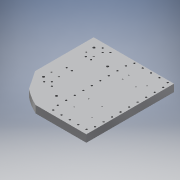
# Autodesk Inventor part: Base Plate Mk 2
Saved by Autodesk Inventor 2017 (Build 210142000, 142)
## iProperties
Created: 2016-12-06
Part Number: Base Plate Mk 2
Material: Aluminum 6061
Document SubType Name: Modeling
Designer: qupec
Density: 2.7 g/cm^3
Appearance: Aluminum - Flat
Mass: 681.535 g
Surface Area: 529.714 cm^2
Volume: 252.42 cm^3
Author: qupec
Autodesk Inventor part; units mm, degrees
ref_plane "YZ Plane" through (0, 0, 0) normal (1, 0, 0) x (0, 1, 0)
ref_plane "XZ Plane" through (0, 0, 0) normal (0, 1, 0) x (-1, 0, 0)
ref_plane "XY Plane" through (0, 0, 0) normal (0, 0, 1) x (1, 0, 0)
sketch "Sketch1" plane through (0, 0, 0) normal (0, 1, 0) x (-1, 0, 0)
  line L0 (69.85, 76.2) -> (-69.85, 76.2)
  line L1 (-69.85, 76.2) -> (-69.85, -76.2)
  line L2 (-69.85, -76.2) -> (69.85, -76.2)
  line L3 (69.85, -76.2) -> (69.85, 76.2)
  point P0 (0, 0)
  dimension "d0" = 152.4
  dimension "d1" = 139.7
  dimension "d2" = 69.85
  dimension "d3" = 76.2
  constraints: 8 end point, 2 parallel, 1 horizontal, 1 perpendicular
  measures "d0" distance of L2.end L0.start
  measures "d1" distance of L0.start L0.end
  measures "d2" distance from line of point (0, 0) L1
  measures "d3" distance from line of point (0, 0) L0
extrude "Extrusion1" add sketch "Sketch1" along normal blind 12.7
fillet "Fillet1" [suppressed]
sketch "Sketch7" plane through (0, 12.7, 0) normal (0, 1, 0) x (1, 0, 0)
  arc A0 (-69.85, -37.0366) -> (-18.2851, -76.2) centre (46.0045, 61.976) ccw
  line L0 (69.85, 76.2) -> (-69.85, 76.2) projected
  line L1 (69.85, -76.2) -> (69.85, 76.2) projected
  line L2 (-69.85, 76.2) -> (-69.85, -76.2) projected
  line L3 (-69.85, -76.2) -> (69.85, -76.2) projected
  line L4 (-69.85, 76.2) -> (-69.85, -76.2) projected
  arc A1 (-18.2851, -76.2) -> (-69.85, -37.0366) centre (46.0045, 61.976) ccw
  point P0 (0, 0)
  point P1 (76.2, -60.325)
  point P2 (73.025, -60.325)
  point P3 (73.025, 63.5)
  point P4 (73.025, 60.325)
  point P5 (-73.025, 63.5)
  point P6 (76.2, 60.325)
  point P7 (73.025, -63.5)
  point P8 (-76.2, 60.325)
  point P9 (-80.9955, -22.2663)
  dimension "d46" = 304.8
  dimension "d47" = 14.224
  dimension "d48" = 23.8455
  constraints: 5 point on circle, 2 centre point, 7 other
  measures "d46" diameter of A0
sketch "Sketch8" plane through (0, 12.7, 0) normal (0, 1, 0) x (1, 0, 0)
  circle A0 centre (-47.526, 7.0319) radius 1.4224 projected
  circle A1 centre (-47.526, 7.0319) radius 1.4224 projected
  circle A2 centre (-38.506, 7.0319) radius 1.4224 projected
  line L0 (-33.996, 3.9778) -> (-52.036, 3.9778) projected
  line L1 (-33.996, 10.086) -> (-33.996, 3.9778) projected
  line L2 (-33.996, 10.086) -> (-52.036, 10.086) projected
  line L3 (-52.036, 3.9778) -> (-52.036, 10.086) projected
  circle A3 centre (-47.526, 40.2937) radius 1.4224 projected
  circle A4 centre (-38.506, 40.2937) radius 1.4224 projected
  line L4 (-33.996, 37.2396) -> (-52.036, 37.2396) projected
  line L5 (-33.996, 43.3478) -> (-33.996, 37.2396) projected
  line L6 (-33.996, 43.3478) -> (-52.036, 43.3478) projected
  line L7 (-52.036, 37.2396) -> (-52.036, 43.3478) projected
  circle A5 centre (2.54, -39.6875) radius 3.175 construction
  circle A6 centre (2.54, 12.7127) radius 3.175 construction
  circle A7 centre (2.54, 65.1129) radius 3.175 construction
  circle A8 centre (68.58, 65.1129) radius 3.175 construction
  circle A9 centre (68.58, 12.7127) radius 3.175 construction
  circle A10 centre (68.58, -39.6875) radius 3.175 construction
  circle A11 centre (-32.4275, -33.782) radius 1.4224 projected
  circle A12 centre (-39.1585, -27.051) radius 1.4224 projected
  circle A13 centre (-45.8895, -33.782) radius 1.4224 projected
  circle A14 centre (-45.8895, 67.818) radius 1.4224 projected
  circle A15 centre (-39.1585, 61.087) radius 1.4224 projected
  circle A16 centre (-32.4275, 67.818) radius 1.4224 projected
extrude "Extrusion9" cut sketch "Sketch8" against normal through all contours A0 | A2 | A3 | A4 | A11 | A12 | A13 | A14 | A15 | A16
extrude "Extrusion11" cut sketch "Sketch7" against normal through all contours A0 L3 L2
sketch "Sketch10" plane through (0, 12.7, 0) normal (0, 1, 0) x (1, 0, 0)
  circle A0 centre (62.611, 72.39) radius 1.4732 projected
  arc A1 (-69.85, -37.0366) -> (-18.2851, -76.2) centre (46.0045, 61.976) ccw projected
  line L0 (-18.2851, -76.2) -> (69.85, -76.2) projected
  line L1 (69.85, -76.2) -> (69.85, 76.2) projected
  line L2 (69.85, 76.2) -> (-69.85, 76.2) projected
  line L3 (-69.85, 76.2) -> (-69.85, -37.0366) projected
  circle A2 centre (-47.526, 40.2937) radius 1.4224 projected
  circle A3 centre (-47.526, 7.0319) radius 1.4224 projected
  circle A4 centre (-38.506, 7.0319) radius 1.4224 projected
  circle A5 centre (-38.506, 40.2937) radius 1.4224 projected
  circle A6 centre (33.655, 72.39) radius 1.4732 projected
  circle A7 centre (48.133, 72.39) radius 1.4732 projected
  circle A8 centre (19.177, 72.39) radius 1.4732 projected
  circle A9 centre (4.699, 72.39) radius 1.4732 projected
  circle A10 centre (62.611, -68.58) radius 1.4732 projected
  circle A11 centre (48.133, -68.58) radius 1.4732 projected
  circle A12 centre (33.655, -68.58) radius 1.4732 projected
  circle A13 centre (19.177, -68.58) radius 1.4732 projected
  circle A14 centre (4.699, -68.58) radius 1.4732 projected
  point P0 (0, 0)
extrude "Extrusion13" cut sketch "Sketch10" against normal through all contours A0 | A6 | A7 | A8 | A9 | A10 | A11 | A12 | A13 | A14
sketch "Sketch11" plane through (0, 12.7, 0) normal (0, 1, 0) x (1, 0, 0)
  circle A0 centre (19.177, 72.39) radius 1.4732 projected
  circle A1 centre (48.133, 72.39) radius 1.4732 projected
  circle A2 centre (62.611, -68.58) radius 1.4732 projected
  circle A3 centre (33.655, -68.58) radius 1.4732 projected
  circle A4 centre (4.699, -68.58) radius 1.4732 projected
  circle A5 centre (1.27, -42.545) radius 1.4732 projected
  circle A6 centre (1.27, -12.9117) radius 1.4732 projected
  circle A7 centre (1.27, 16.7217) radius 1.4732 projected
  circle A8 centre (1.27, 46.355) radius 1.4732 projected
  circle A9 centre (66.04, 61.1717) radius 1.4732 projected
  circle A10 centre (66.04, 31.5383) radius 1.4732 projected
  circle A11 centre (66.04, 1.905) radius 1.4732 projected
  circle A12 centre (66.04, -27.7283) radius 1.4732 projected
  circle A13 centre (66.04, -57.3617) radius 1.4732 projected
  circle A14 centre (66.04, -42.545) radius 1.4732 projected
  circle A15 centre (66.04, -12.9117) radius 1.4732 projected
  circle A16 centre (66.04, 16.7217) radius 1.4732 projected
  circle A17 centre (66.04, 46.355) radius 1.4732 projected
  circle A18 centre (1.27, 61.1717) radius 1.4732 projected
  circle A19 centre (1.27, 31.5383) radius 1.4732 projected
  circle A20 centre (1.27, 1.905) radius 1.4732 projected
  circle A21 centre (1.27, -27.7283) radius 1.4732 projected
  circle A22 centre (1.27, -57.3617) radius 1.4732 projected
  circle A23 centre (19.177, -68.58) radius 1.4732 projected
  circle A24 centre (48.133, -68.58) radius 1.4732 projected
  circle A25 centre (62.611, 72.39) radius 1.4732 projected
  circle A26 centre (33.655, 72.39) radius 1.4732 projected
  circle A27 centre (4.699, 72.39) radius 1.4732 projected
  line L0 (0.635, -72.39) -> (66.675, -72.39) projected
  line L1 (69.85, -69.215) -> (69.85, 73.025) projected
  line L2 (66.675, 76.2) -> (0.635, 76.2) projected
  line L3 (-2.54, 73.025) -> (-2.54, -69.215) projected
  arc A28 (59.055, 62.23) -> (55.88, 65.405) centre (55.88, 62.23) ccw projected
  line L4 (59.055, -58.42) -> (59.055, 62.23) projected
  arc A29 (55.88, -61.595) -> (59.055, -58.42) centre (55.88, -58.42) ccw projected
  line L5 (11.43, -61.595) -> (55.88, -61.595) projected
  arc A30 (8.255, -58.42) -> (11.43, -61.595) centre (11.43, -58.42) ccw projected
  line L6 (8.255, 62.23) -> (8.255, -58.42) projected
  arc A31 (11.43, 65.405) -> (8.255, 62.23) centre (11.43, 62.23) ccw projected
  line L7 (55.88, 65.405) -> (11.43, 65.405) projected
  arc A32 (69.85, 73.025) -> (66.675, 76.2) centre (66.675, 73.025) ccw projected
  arc A33 (0.635, 76.2) -> (-2.54, 73.025) centre (0.635, 73.025) ccw projected
  arc A34 (-2.54, -69.215) -> (0.635, -72.39) centre (0.635, -69.215) ccw projected
  arc A35 (66.675, -72.39) -> (69.85, -69.215) centre (66.675, -69.215) ccw projected
  point P0 (0, 0)
  point P1 (52.705, -61.595)
extrude "Extrusion14" cut sketch "Sketch11" against normal through all contours A5 | A6 | A7 | A8 | A9 | A10 | A11 | A12 | A13 | A14 | A15 | A16 | A17 | A18 | A19 | A20 | A21 | A22 | A25
sketch "Sketch14" plane through (0, 0, 0) normal (0, -1, 0) x (1, 0, 0)
  line L0 (69.85, -76.2) -> (-69.85, -76.2) projected
  line L1 (-18.2851, 76.2) -> (69.85, 76.2) projected
  circle A0 centre (4.699, -72.39) radius 1.4732 projected
  circle A1 centre (-32.4275, -67.818) radius 1.4224 projected
  point P0 (0, 0)
  point P1 (-13.8643, 44.45)
  point P2 (-13.8643, -44.45)
  dimension "d79" = 44.45
  dimension "d80" = 152.4
  dimension "d81" = 44.45
  dimension "d82" = 37.1265
  dimension "d83" = 18.5633
  dimension "d84" = 18.5633
  measures "d79" vertical distance of point (0, 0) point (-13.864, 44.45)
  measures "d80" distance between parallel lines of L0 L1
  measures "d81" vertical distance of point (-13.864, -44.45) point (0, 0)
  measures "d82" horizontal distance of A0.centre A1.centre
  measures "d83" horizontal distance of A1.centre point (-13.864, -44.45)
  measures "d84" horizontal distance of A1.centre point (-13.864, 44.45)
hole "Hole2" at (-13.8643, 0, 44.45) at (-13.8643, 0, -44.45) direction (0, 1, 0) diameter 3.9624 end through all thread size "10-32 UNF" class "2B" standard "ANSI Unified Screw Threads"
sketch "Sketch15" plane through (0, 0, 0) normal (0, -1, 0) x (1, 0, 0)
  circle A0 centre (-13.8643, 44.45) radius 1.9812 projected
  circle A1 centre (-13.8643, -44.45) radius 1.9812 projected
  circle A2 centre (66.04, -31.5383) radius 1.4732 projected
  circle A3 centre (1.27, -31.5383) radius 1.4732 projected
  circle A4 centre (1.27, 42.545) radius 1.4732 projected
  point P0 (0, 0)
  point P1 (33.655, -44.45)
  point P2 (33.655, 44.45)
  point P3 (33.655, 0)
  dimension "d92" = 44.45
  dimension "d93" = 44.45
  dimension "d94" = 44.45
  dimension "d95" = 44.45
  dimension "d96" = 64.77
  dimension "d97" = 32.385
  dimension "d98" = 32.385
  dimension "d222" = 32.385
  dimension "d223" = 44.45
  measures "d92" vertical distance of point (0, 0) point (33.655, 44.45)
  measures "d93" vertical distance of point (0, 0) A0.centre
  measures "d94" vertical distance of point (0, 0) A1.centre
  measures "d95" vertical distance of point (33.655, -44.45) point (0, 0)
  measures "d96" distance between centres of A2 A3
  measures "d97" horizontal distance of A3.centre point (33.655, -44.45)
  measures "d98" horizontal distance of point (33.655, 44.45) A4.centre
  measures "d222" horizontal distance of A4.centre point (33.655, 0)
  measures "d223" distance of point (33.655, -44.45) point (33.655, 0)
hole "Hole3" at (33.655, 0, -44.45) at (33.655, 0, 44.45) at (33.655, 0, 0) direction (0, 1, 0) diameter 3.9624 depth 9.525 thread size "10-32 UNF" class "2B" standard "ANSI Unified Screw Threads"
thread "Thread3" size "5-40 UNC" class "2B" standard "ANSI Unified Screw Threads" full length
thread "Thread4" size "5-40 UNC" class "2B" standard "ANSI Unified Screw Threads" full length
thread "Thread5" size "5-40 UNC" class "2B" standard "ANSI Unified Screw Threads" full length
thread "Thread6" size "5-40 UNC" class "2B" standard "ANSI Unified Screw Threads" full length
thread "Thread7" size "5-40 UNC" class "2B" standard "ANSI Unified Screw Threads" full length
thread "Thread8" size "5-40 UNC" class "2B" standard "ANSI Unified Screw Threads" full length
thread "Thread9" size "5-40 UNC" class "2B" standard "ANSI Unified Screw Threads" full length
thread "Thread10" size "5-40 UNC" class "2B" standard "ANSI Unified Screw Threads" full length
thread "Thread11" size "5-40 UNC" class "2B" standard "ANSI Unified Screw Threads" full length
thread "Thread12" size "5-40 UNC" class "2B" standard "ANSI Unified Screw Threads" full length
thread "Thread13" size "5-40 UNC" class "2B" standard "ANSI Unified Screw Threads" full length
thread "Thread14" size "5-40 UNC" class "2B" standard "ANSI Unified Screw Threads" full length
thread "Thread15" size "5-40 UNC" class "2B" standard "ANSI Unified Screw Threads" full length
thread "Thread16" size "5-40 UNC" class "2B" standard "ANSI Unified Screw Threads" full length
thread "Thread17" size "5-40 UNC" class "2B" standard "ANSI Unified Screw Threads" full length
thread "Thread18" size "5-40 UNC" class "2B" standard "ANSI Unified Screw Threads" full length
thread "Thread19" size "5-40 UNC" class "2B" standard "ANSI Unified Screw Threads" full length
thread "Thread20" size "5-40 UNC" class "2B" standard "ANSI Unified Screw Threads" full length
thread "Thread21" size "5-40 UNC" class "2B" standard "ANSI Unified Screw Threads" full length
thread "Thread22" size "5-40 UNC" class "2B" standard "ANSI Unified Screw Threads" full length
thread "Thread23" size "5-40 UNC" class "2B" standard "ANSI Unified Screw Threads" full length
thread "Thread24" size "5-40 UNC" class "2B" standard "ANSI Unified Screw Threads" full length
thread "Thread25" size "5-40 UNC" class "2B" standard "ANSI Unified Screw Threads" full length
thread "Thread26" size "5-40 UNC" class "2B" standard "ANSI Unified Screw Threads" full length
thread "Thread27" size "5-40 UNC" class "2B" standard "ANSI Unified Screw Threads" full length
thread "Thread28" size "5-40 UNC" class "2B" standard "ANSI Unified Screw Threads" full length
thread "Thread29" size "5-40 UNC" class "2B" standard "ANSI Unified Screw Threads" full length
thread "Thread30" size "5-40 UNC" class "2B" standard "ANSI Unified Screw Threads" full length
thread "Thread31" size "5-40 UNC" class "2B" standard "ANSI Unified Screw Threads" full length
thread "Thread32" size "4-40 UNC" class "2B" standard "ANSI Unified Screw Threads" full length
thread "Thread33" size "4-40 UNC" class "2B" standard "ANSI Unified Screw Threads" full length
thread "Thread34" size "4-40 UNC" class "2B" standard "ANSI Unified Screw Threads" full length
thread "Thread35" size "4-40 UNC" class "2B" standard "ANSI Unified Screw Threads" full length
thread "Thread36" size "4-40 UNC" class "2B" standard "ANSI Unified Screw Threads" full length
thread "Thread37" size "4-40 UNC" class "2B" standard "ANSI Unified Screw Threads" full length
thread "Thread38" size "4-40 UNC" class "2B" standard "ANSI Unified Screw Threads" full length
thread "Thread39" size "4-40 UNC" class "2B" standard "ANSI Unified Screw Threads" full length
thread "Thread40" size "4-40 UNC" class "2B" standard "ANSI Unified Screw Threads" full length
thread "Thread41" size "4-40 UNC" class "2B" standard "ANSI Unified Screw Threads" full length
sketch "Sketch17" plane through (0, 12.7, 0) normal (0, 1, 0) x (1, 0, 0)
  line L0 (-48.26, -57.7736) -> (-69.85, -25.6538)
  line L1 (-69.85, 76.2) -> (-69.85, -37.0366) projected
  line L2 (-69.85, -25.6538) -> (-69.85, -37.0366)
  arc A0 (-69.85, -37.0366) -> (-18.2851, -76.2) centre (46.0045, 61.976) ccw projected
  arc A1 (-69.85, -37.0366) -> (-48.26, -57.7736) centre (46.0045, 61.976) ccw
  point P0 (0, 0)
  dimension "d200" = 6.35
  dimension "d203" = 21.59
  constraints: 4 end point, 3 point on circle, 1 centre point, 1 concentric, 1 point on line
  measures "d200" distance from line of L1.end L0
  measures "d203" horizontal distance of L1.end L0.start
extrude "Extrusion16" cut sketch "Sketch17" against normal through all
thread "Thread46" size "10-32 UNF" class "2B" standard "ANSI Unified Screw Threads" full length
thread "Thread47" size "10-32 UNF" class "2B" standard "ANSI Unified Screw Threads" full length
thread "Thread48" size "10-32 UNF" class "2B" standard "ANSI Unified Screw Threads" full length
sketch "Sketch19" plane through (0, 12.7, 0) normal (0, 1, 0) x (1, 0, 0)
  circle A0 centre (49.53, 49.53) radius 1.025
  line L0 (-18.2851, -76.2) -> (69.85, -76.2) projected
  line L1 (69.85, -76.2) -> (69.85, 76.2) projected
  line L2 (69.85, 76.2) -> (-69.85, 76.2) projected
  circle A1 centre (49.53, -45.72) radius 1.025
  circle A2 centre (17.78, 49.53) radius 1.025
  circle A3 centre (17.78, -45.72) radius 1.025
  circle A4 centre (18.415, -20.745) radius 1.0287
  circle A5 centre (18.415, 38.255) radius 1.0287
  circle A6 centre (41.415, -20.745) radius 1.0287
  circle A7 centre (41.415, 38.255) radius 1.0287
  point P0 (0, 0)
  point P1 (-28.9602, -57.9611)
  point P2 (18.415, 8.255)
  dimension "d239" = 2.05
  dimension "d241" = 20.32
  dimension "d242" = 26.67
  dimension "d245" = 95.25
  dimension "d248" = 31.75
  dimension "d251" = 31.115
  dimension "d252" = 53.975
  dimension "d253" = 2.0574
  dimension "d254" = 29
  dimension "d257" = 59
  dimension "d260" = 23
  constraints: 8 centre point, 2 horizontal, 2 vertical, 12 other
  measures "d239" diameter of A0
  measures "d241" distance from line of L1 A0.centre
  measures "d242" distance from line of A0.centre L2
  measures "d245" distance of A0.centre A1.centre
  measures "d248" distance of A0.centre A2.centre
  measures "d251" horizontal distance of point (18.415, 8.255) A1.centre
  measures "d252" vertical distance of A1.centre point (18.415, 8.255)
  measures "d253" diameter of A4
  measures "d254" distance of point (18.415, 8.255) A4.centre
  measures "d257" distance of A4.centre A5.centre
  measures "d260" distance of A4.centre A6.centre
sketch "Sketch18" plane through (0, 12.7, 0) normal (0, 1, 0) x (1, 0, 0)
  circle A0 centre (-47.6269, -14.097) radius 2.794 projected
  circle A1 centre (-47.6269, 48.133) radius 2.794 projected
  point P0 (0, 0)
  point P1 (-53.9769, 60.833)
  point P2 (-53.9769, -26.797)
  dimension "d211" = 12.7
  dimension "d212" = 12.7
  dimension "d213" = 6.35
  dimension "d214" = 6.35
  measures "d211" vertical distance of A0.centre point (-53.977, -26.797)
  measures "d212" vertical distance of A1.centre point (-53.977, 60.833)
  measures "d213" horizontal distance of A1.centre point (-53.977, 60.833)
  measures "d214" horizontal distance of A0.centre point (-53.977, -26.797)
hole "Hole4" at (-53.9769, 12.7, -60.833) at (-53.9769, 12.7, 26.797) direction (0, -1, 0) diameter 3.9624 depth 12.7 thread size "10-32 UNF" class "2B" standard "ANSI Unified Screw Threads"
sketch "Sketch21" plane through (0, 12.7, 0) normal (0, 1, 0) x (1, 0, 0)
  line L0 (69.85, 76.2) -> (-69.85, 76.2) projected
  line L1 (-69.85, 76.2) -> (-69.85, -25.6538) projected
  point P0 (0, 0)
  point P1 (-53.9242, -13.1826)
  point P2 (-40.9194, -13.1826)
  point P3 (-40.9194, 47.1932)
  point P4 (-53.9242, 47.1932)
  dimension "d224" = 29.0068
  dimension "d225" = 15.9258
  dimension "d226" = 28.9306
  dimension "d227" = 29.0068
  dimension "d228" = 15.9258
  dimension "d229" = 89.3826
  dimension "d230" = 89.3826
  dimension "d231" = 28.9306
  measures "d224" distance from line of L0 point (-53.924, 47.193)
  measures "d225" distance from line of point (-53.924, 47.193) L1
  measures "d226" distance from line of L1 point (-40.919, 47.193)
  measures "d227" distance from line of L0 point (-40.919, 47.193)
  measures "d228" distance from line of L1 point (-53.924, -13.183)
  measures "d229" distance from line of L0 point (-53.924, -13.183)
  measures "d230" distance from line of L0 point (-40.919, -13.183)
  measures "d231" distance from line of L1 point (-40.919, -13.183)
hole "Hole5" at (-53.9242, 12.7, 13.1826) at (-40.9194, 12.7, 13.1826) at (-53.9242, 12.7, -47.1932) at (-40.9194, 12.7, -47.1932) direction (0, -1, 0) diameter 2.8448 end through all
extrude "Extrusion17" cut sketch "Sketch19" against normal blind 5.08
equation "\"d2\" = 0.5 * d1"
equation "\"d3\" = 0.5 * d0"
equation "\"d79\" = d81"
equation "\"d83\" = 0.5 * d82"
equation "\"d84\" = d83"
equation "\"d92\" = d93"
equation "\"d95\" = d94"
equation "\"d97\" = 0.5 * d96"
equation "\"d98\" = d97"
equation "\"d222\" = d98"
equation "\"d223\" = d95"
equation "\"d214\" = d213"
equation "\"d227\" = d224"
equation "\"d228\" = d225"
equation "\"d230\" = d229"
equation "\"d231\" = d226"
body "Solid1"
